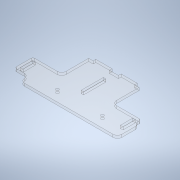
# Autodesk Inventor part: trackingCamMountFront
Saved by Autodesk Inventor 2020 (Build 240168000, 168)
## iProperties
Created: 2020-03-02
Part Number: trackingCamMountFront
Material: Polycarbonate, Clear
Document SubType Name: Modeling
Designer: n10208577
Density: 1.2 g/cm^3
Appearance: Polycarbonate - Clear
Author: n10208577
Autodesk Inventor part; units mm, degrees
ref_plane "YZ Plane" through (0, 0, 0) normal (1, 0, 0) x (0, 1, 0)
ref_plane "XZ Plane" through (0, 0, 0) normal (0, 1, 0) x (-1, 0, 0)
ref_plane "XY Plane" through (0, 0, 0) normal (0, 0, 1) x (1, 0, 0)
sketch "Sketch1" plane through (0, 0, 0) normal (0, 1, 0) x (-1, 0, 0)
  line L0 (63.3757, -1.1026) -> (45.3757, -1.1026)
  line L1 (73.3757, -1.1026) -> (91.3757, -1.1026)
  line L2 (63.3757, 1.8974) -> (63.3757, -1.1026)
  line L3 (45.3757, -1.1026) -> (45.3757, 1.8974)
  line L4 (73.3757, 1.8974) -> (73.3757, -1.1026)
  line L5 (91.3757, 1.8974) -> (91.3757, -1.1026)
  line L6 (63.3757, 1.8974) -> (73.3757, 1.8974)
  line L7 (45.3757, 1.8974) -> (40.3757, 1.8974)
  line L8 (91.3757, 1.8974) -> (96.3757, 1.8974)
  circle A0 centre (33.8757, 49.1474) radius 1.6
  circle A1 centre (83.8757, 49.1474) radius 1.6
  line L9 (9.8757, 61.3974) -> (107.8757, 61.3974)
  arc A2 (112.8694, 56.6474) -> (107.8757, 61.3974) centre (107.8757, 56.3974) ccw
  arc A3 (112.8694, 56.6474) -> (117.8632, 51.8974) centre (117.8632, 56.8974) ccw
  arc A4 (4.8757, 41.8974) -> (7.3757, 37.5673) centre (9.8757, 41.8974) ccw
  arc A5 (8.3757, 35.8353) -> (7.3757, 37.5673) centre (6.3757, 35.8353) ccw
  line L10 (4.8757, 56.3974) -> (4.8757, 41.8974)
  arc A6 (9.8757, 61.3974) -> (4.8757, 56.3974) centre (9.8757, 56.3974) ccw
  line L11 (96.3757, 1.8974) -> (96.3757, 26.8974)
  line L12 (66.9757, 12.1474) -> (66.9757, 36.8474)
  line L13 (69.7757, 36.8474) -> (69.7757, 12.1474)
  line L14 (69.7757, 36.8474) -> (66.9757, 36.8474)
  line L15 (69.7757, 12.1474) -> (66.9757, 12.1474)
  line L16 (40.3757, 1.8974) -> (40.3757, 26.8974)
  arc A7 (40.3757, 26.8974) -> (35.3757, 31.8974) centre (35.3757, 26.8974) ccw
  line L17 (14.3757, 48.7474) -> (14.3757, 35.0474)
  line L18 (11.3757, 35.0474) -> (14.3757, 35.0474)
  line L19 (11.3757, 48.7474) -> (14.3757, 48.7474)
  line L20 (11.3757, 48.7474) -> (11.3757, 35.0474)
  line L21 (10.3757, 31.8974) -> (35.3757, 31.8974)
  arc A8 (8.3757, 33.8974) -> (10.3757, 31.8974) centre (10.3757, 33.8974) ccw
  line L22 (122.3757, 48.7474) -> (122.3757, 35.0474)
  line L23 (125.3757, 35.0474) -> (122.3757, 35.0474)
  line L24 (125.3757, 48.7474) -> (122.3757, 48.7474)
  line L25 (125.3757, 48.7474) -> (125.3757, 35.0474)
  line L26 (101.3757, 31.8974) -> (126.3757, 31.8974)
  arc A9 (101.3757, 31.8974) -> (96.3757, 26.8974) centre (101.3757, 26.8974) ccw
  line L27 (128.3757, 33.8974) -> (128.3757, 49.8974)
  arc A10 (126.3757, 31.8974) -> (128.3757, 33.8974) centre (126.3757, 33.8974) ccw
  arc A11 (128.3757, 49.8974) -> (126.3757, 51.8974) centre (126.3757, 49.8974) ccw
  line L28 (126.3757, 51.8974) -> (117.8632, 51.8974)
  line L29 (8.3757, 33.8974) -> (8.3757, 35.8353)
  constraints: 60 end point, 20 point on circle, 12 centre point
extrude "Extrusion1" add sketch "Sketch1" along normal blind 3
body "Solid1"
